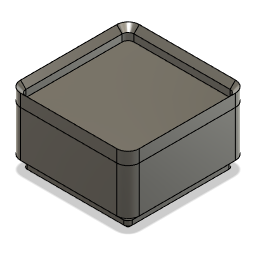
Gridfinity template (Autodesk Fusion 360 design; units mm, degrees)
Autodesk Fusion 360 part; units mm, degrees
sketch "Main body" plane through (0, 0, 0) normal (0, 1, 0) x (1, 0, 0)
  line L0 (-4, 0) -> (-38, 0)
  line L1 (-42, -4) -> (-42, -38)
  line L2 (-38, -42) -> (-4, -42)
  line L3 (0, -38) -> (0, -4)
  arc A0 (-4, -42) -> (0, -38) centre (-4, -38) ccw
  arc A1 (-42, -38) -> (-38, -42) centre (-38, -38) ccw
  arc A2 (-38, 0) -> (-42, -4) centre (-38, -4) ccw
  arc A3 (0, -4) -> (-4, 0) centre (-4, -4) ccw
  point P0 (-42, 0)
  point P1 (0, -42)
  dimension "d1" = 42
  dimension "d2" = 42
  dimension "d4" = 4
  constraint horizontal L0
  constraint vertical L1
  constraint horizontal L2
  constraint vertical L3
  constraint coincident P1 L2
  constraint coincident P1 L3
  constraint tangent L2 A0
  constraint tangent L3 A0
  constraint tangent L1 A1
  constraint tangent L2 A1
  constraint equal A0 A1
  constraint coincident P0 L0
  constraint coincident P0 L1
  constraint tangent L0 A2
  constraint tangent L1 A2
  constraint equal A0 A2
  constraint coincident origin L0
  constraint coincident origin L3
  constraint tangent L0 A3
  constraint tangent L3 A3
  constraint equal A0 A3
  measures "d1" distance of origin P0
  measures "d2" distance of origin P1
  measures "d4" radius of A0
sketch "Leg" plane through (0, 0, 0) normal (0, 1, 0) x (1, 0, 0)
  line L0 (-3.9, -39.6) -> (-38.1, -39.6)
  line L1 (-39.6, -38.1) -> (-39.6, -3.9)
  line L2 (-38.1, -2.4) -> (-3.9, -2.4)
  line L3 (-2.4, -3.9) -> (-2.4, -38.1)
  line L4 (-38, -42) -> (-4, -42)
  line L5 (-42, -4) -> (-42, -38)
  line L6 (0, -38) -> (0, -4)
  line L7 (-4, 0) -> (-38, 0)
  arc A0 (-39.6, -38.1) -> (-38.1, -39.6) centre (-38.1, -38.1) ccw
  arc A1 (-3.9, -39.6) -> (-2.4, -38.1) centre (-3.9, -38.1) ccw
  arc A2 (-2.4, -3.9) -> (-3.9, -2.4) centre (-3.9, -3.9) ccw
  arc A3 (-38.1, -2.4) -> (-39.6, -3.9) centre (-38.1, -3.9) ccw
  circle A4 centre (-8, -34) radius 1.5
  circle A5 centre (-8, -34) radius 3.25
  circle A6 centre (-34, -34) radius 3.25
  circle A7 centre (-34, -34) radius 1.5
  circle A8 centre (-8, -8) radius 3.25
  circle A9 centre (-8, -8) radius 1.5
  circle A10 centre (-34, -8) radius 3.25
  circle A11 centre (-34, -8) radius 1.5
  point P0 (-2.4, -39.6)
  point P1 (-39.6, -39.6)
  point P2 (-2.4, -2.4)
  dimension "d7" = 37.2
  dimension "d8" = 37.2
  dimension "d9" = 1.5
  dimension "d12" = 3
  dimension "d13" = 6.5
  dimension "d24" = 2.4
  dimension "d25" = 2.4
  dimension "d26" = 5.6
  dimension "d27" = 5.6
  dimension "d28" = 5.6
  dimension "d29" = 5.6
  dimension "d30" = 5.6
  dimension "d31" = 5.6
  dimension "d32" = 5.6
  dimension "d33" = 5.6
  constraint horizontal L0
  constraint vertical L1
  constraint horizontal L2
  constraint vertical L3
  constraint coincident P1 L0
  constraint coincident P1 L1
  constraint tangent L0 A0
  constraint tangent L1 A0
  constraint coincident P0 L0
  constraint coincident P0 L3
  constraint tangent L0 A1
  constraint tangent L3 A1
  constraint equal A0 A1
  constraint coincident P2 L2
  constraint coincident P2 L3
  constraint tangent L2 A2
  constraint tangent L3 A2
  constraint equal A0 A2
  constraint tangent L1 A3
  constraint tangent L2 A3
  constraint equal A0 A3
  constraint concentric A4 A5
  constraint concentric A6 A7
  constraint concentric A10 A11
  constraint concentric A8 A9
  measures "d7" distance of P0 P1
  measures "d8" distance of P0 P2
  measures "d9" radius of A0
  measures "d12" diameter of A4
  measures "d13" diameter of A5
  measures "d24" distance of L1 L5
  measures "d25" distance of L0 L4
  measures "d26" distance of L0 A4.centre
  measures "d27" distance of L3 A4.centre
  measures "d28" distance of L1 A6.centre
  measures "d29" distance of L0 A6.centre
  measures "d30" distance of L1 A10.centre
  measures "d31" distance of L2 A10.centre
  measures "d32" distance of L3 A8.centre
  measures "d33" distance of L2 A8.centre
sketch "Leg to body transition" plane through (0, 0, 0) normal (0, 1, 0) x (1, 0, 0)
  line L0 (-4, -42) -> (-38, -42)
  line L1 (-42, -38) -> (-42, -4)
  line L2 (-38, 0) -> (-4, 0)
  line L3 (0, -4) -> (0, -38)
  arc A0 (-42, -38) -> (-38, -42) centre (-38, -38) ccw
  arc A1 (-4, -42) -> (0, -38) centre (-4, -38) ccw
  arc A2 (0, -4) -> (-4, 0) centre (-4, -4) ccw
  arc A3 (-38, 0) -> (-42, -4) centre (-38, -4) ccw
  line L4 (-3.9, -39.6) -> (-38.1, -39.6)
  line L5 (-2.4, -3.9) -> (-2.4, -38.1)
  line L6 (-39.6, -38.1) -> (-39.6, -3.9)
  line L7 (-38.1, -2.4) -> (-3.9, -2.4)
  circle A4 centre (-8, -34) radius 1.5
  circle A5 centre (-34, -34) radius 1.5
  circle A6 centre (-34, -8) radius 1.5
  circle A7 centre (-8, -8) radius 1.5
  point P0 (0, -42)
  point P1 (-42, 0)
  dimension "d54" = 4
  dimension "d55" = 2.4
  dimension "d56" = 2.4
  dimension "d57" = 2.4
  dimension "d58" = 2.4
  constraint horizontal L0
  constraint vertical L1
  constraint horizontal L2
  constraint vertical L3
  constraint tangent L0 A0
  constraint tangent L1 A0
  constraint tangent L0 A1
  constraint tangent L3 A1
  constraint equal A0 A1
  constraint tangent L2 A2
  constraint tangent L3 A2
  constraint equal A0 A2
  constraint tangent L1 A3
  constraint tangent L2 A3
  constraint equal A0 A3
  measures "d54" radius of A0
  measures "d55" distance of L0 L4
  measures "d56" distance of L1 L6
  measures "d57" distance of L2 L7
  measures "d58" distance of L3 L5
extrude "Extrude1" add sketch "Leg" against normal blind 2.6 contours L0 L1 L2 L3 A0 A1 A2 A3 makes body 1
chamfer "Chamfer2" distance 0.8 angle 45 8 edges at (-39.6, -2.6, 21) (-39.1607, -2.6, 2.8393) (-21, -2.6, 2.4) (-2.8393, -2.6, 2.8393) (-2.4, -2.6, 21) (-2.8393, -2.6, 39.1607) (-21, -2.6, 39.6) (-39.1607, -2.6, 39.1607) on bodies 1
extrude "Extrude6" add sketch "Leg to body transition" along normal blind 2.15 bodies 1
chamfer "Chamfer5" distance 2.15 angle 45 8 edges at (-21, 0, 0) (-1.1716, 0, 1.1716) (0, 0, 21) (-1.1716, 0, 40.8284) (-21, 0, 42) (-40.8284, 0, 40.8284) (-42, 0, 21) (-40.8284, 0, 1.1716) on bodies 1
extrude "Extrude3" add sketch "Main body" along normal blind 16.225 separate body makes body 2
move_body "Move1" bodies 2 to x (1, 0, 0) y (0, 1, 0) z (0, 0, 1) at (0, 2.15, 0)
sketch "Crown" plane through (0, 18.375, 0) normal (0, 1, 0) x (-1, 0, 0)
  arc A0 (0, 4) -> (4, 0) centre (4, 4) ccw
  line L0 (4, 0) -> (38, 0)
  arc A1 (38, 0) -> (42, 4) centre (38, 4) ccw
  line L1 (42, 4) -> (42, 38)
  arc A2 (42, 38) -> (38, 42) centre (38, 38) ccw
  line L2 (38, 42) -> (4, 42)
  arc A3 (4, 42) -> (0, 38) centre (4, 38) ccw
  line L3 (0, 38) -> (0, 4)
  line L4 (1.9, 38) -> (1.9, 4)
  arc A4 (1.9, 4) -> (4, 1.9) centre (4, 4) ccw
  line L5 (4, 1.9) -> (38, 1.9)
  arc A5 (38, 1.9) -> (40.1, 4) centre (38, 4) ccw
  line L6 (40.1, 4) -> (40.1, 38)
  arc A6 (40.1, 38) -> (38, 40.1) centre (38, 38) ccw
  line L7 (38, 40.1) -> (4, 40.1)
  arc A7 (4, 40.1) -> (1.9, 38) centre (4, 38) ccw
  dimension "d66" = -1.9
split_face "SplitFace2" 1 faces at (-26.6667, 18.375, 28) by curves path "Crown" along L7 A7 L4 A4 L5 A5 L6 A6 on bodies 2
extrude "Extrude7" add sketch "Crown" along normal blind 4.4 separate body makes body 3
chamfer "Chamfer6" distance 1.9 angle 45 8 edges at (-21, 22.775, 40.1) (-39.4849, 22.775, 39.4849) (-40.1, 22.775, 21) (-39.4849, 22.775, 2.5151) (-21, 22.775, 1.9) (-2.5151, 22.775, 2.5151) (-1.9, 22.775, 21) (-2.5151, 22.775, 39.4849) on bodies 3
pattern_linear "R-Pattern2" count 1 spacing 0 along (0, 0, 1) of bodies 1 merged
equation "d1 = body_size_width"
equation "d2 = body_size_lenght"
equation "Blocks_width = 1" comment "1 width = one column of blocks"
equation "Blocks_lenght = 1" comment "1 lenght = one row of blocks"
equation "Blocks_height = 1 / 2" comment "Height of block; 1/2 is half block and 1 is full block"
equation "body_size_width = ( 42 * Blocks_width ) * 1 mm"
equation "body_size_lenght = ( 42 * Blocks_lenght ) * 1 mm"
equation "d24 = ( ( 42 - 37.20 ) / 2 ) * 1 mm"
equation "d25 = ( ( 42 - 37.20 ) / 2 ) * 1 mm"
equation "body_size_height = ( 42.45 * Blocks_height ) * 1 mm - 5 mm"
equation "d37 = body_size_height"
equation "d48 = Blocks_lenght"
equation "d49 = Blocks_width"
equation "d50 = ( -42 * ( Blocks_lenght - 1 ) ) * 1 mm"
equation "d51 = ( 42 * ( Blocks_width - 1 ) ) * 1 mm"
named bodies: "Leg", "Main body", "Crown"
